łozysko wzdłuzne 55_78_16 v2 (Autodesk Fusion 360 design; units mm, degrees)
Autodesk Fusion 360 part; units mm, degrees
sketch "Sketch1" plane through (0, 0, 0) normal (0, 0, 1) x (1, 0, 0)
  circle A0 centre (0, 0) radius 39
  circle A1 centre (0, 0) radius 27.5
  dimension "d1" = 78
  dimension "d2" = 55
  constraint coincident A0.centre A1.centre
  constraint concentric A0 A1
  measures "d1" diameter of A0
  measures "d2" diameter of A1
extrude "Extrude1" add sketch "Sketch1" along normal blind 5 makes body 1
ref_plane "WorkPlane1" through (0, 0, 11) normal (0, 0, 1) x (1, 0, 0)
sketch "Sketch2" plane through (0, 0, 11) normal (0, 0, 1) x (1, 0, 0)
  circle A0 centre (0, 0) radius 27.5
  circle A1 centre (0, 0) radius 39
extrude "Extrude2" add sketch "Sketch2" along normal blind 5 separate body makes body 2
ref_plane "WorkPlane2" through (0, -39, 14.7739) normal (0, -1, 0) x (-1, 0, 0)
ref_plane "WorkPlane3" through (0, 0, 14.7739) normal (0, -1, 0) x (-1, 0, 0)
sketch "Sketch3" plane through (0, 0, 0) normal (0, -1, 0) x (-1, 0, 0)
  line L0 (-39, -11) -> (39, -11)
  line L1 (-39, -5) -> (39, -5)
  line L2 (27.5, -5) -> (-27.5, -5) construction
  line L3 (27.5, -11) -> (-27.5, -11) construction
  line L4 (27.5, -11) -> (39, -5) construction
  circle A0 centre (33.25, -8) radius 4
  line L5 (0, -11) -> (0, -5) construction
  dimension "d10" = 8
  constraint coincident L3.start L4.start
  constraint coincident L1.end L4.end
  constraint midpoint L4 A0.centre
  constraint midpoint L0 L5.start
  constraint midpoint L1 L5.end
  measures "d10" diameter of A0
revolve "Revolve1" cut sketch "Sketch3" angle 360 about axis through (0, 0, 11) along (0, 0, -1) bodies 1 2
sphere "SpherePrimitive1" add diameter 8 placed x (-1, 0, 0) y (0, 0, -1) z (0, -1, 0) at (-33.2672, 0, 8.0004) separate body makes body 3
pattern_circular "C-Pattern1" count 24 over 360 about axis through (0, 0, 11) along (0, 0, -1) of bodies 3 makes body 4 at (-35.5765, 10.4139, 8.9459) makes body 5 at (-31.6689, 19.2669, 8.9459) makes body 6 at (-25.6032, 26.8069, 8.9459) makes body 7 at (-17.7927, 32.5201, 8.9459) makes body 8 at (-8.7696, 36.0171, 7.0548) makes body 9 at (0.8511, 37.0595, 7.0548) makes body 10 at (10.4139, 35.5765, 8.9459) makes body 11 at (19.2669, 31.6689, 8.9459) makes body 12 at (26.8069, 25.6032, 8.9459) makes body 13 at (32.5201, 17.7927, 7.0548) makes body 14 at (36.0171, 8.7696, 7.0548) makes body 15 at (37.0595, -0.8511, 7.0548) makes body 16 at (35.5765, -10.4139, 7.0548) makes body 17 at (31.6689, -19.2669, 7.0548) makes body 18 at (25.6032, -26.8069, 8.9459) makes body 19 at (17.7927, -32.5201, 7.0548) makes body 20 at (8.7696, -36.0171, 7.0548) makes body 21 at (-0.8511, -37.0595, 7.0548) makes body 22 at (-10.4139, -35.5765, 7.0548) makes body 23 at (-19.2669, -31.6689, 7.0548) makes body 24 at (-26.8069, -25.6032, 8.9459) makes body 25 at (-32.5201, -17.7927, 7.0548) makes body 26 at (-36.0171, -8.7696, 7.0548)
equation "d9 = ( -78 / 2 ) * 1 mm"
